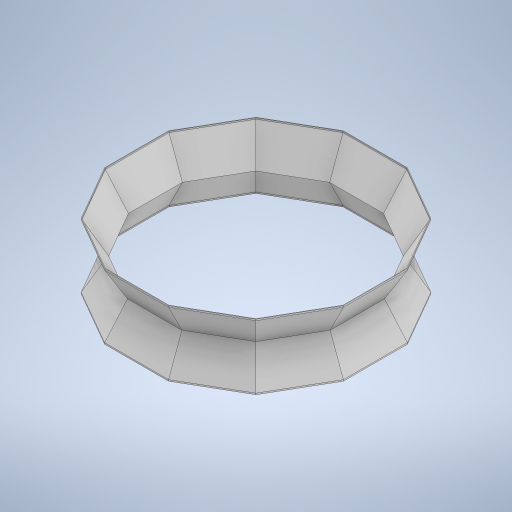
# Autodesk Inventor part: OV-PAM_n_12_standard_1F
Saved by Autodesk Inventor 2024 (Build 280153000, 153)
## iProperties
Created: 2023-08-31
Part Number: OV-PAM_n_12_standard_1F
Material: 일반
Document SubType Name: Modeling
Designer: jsw
Density: 1 g/cm^3
Appearance: 기본값
Author: jsw
Autodesk Inventor part; units mm, degrees
ref_plane "YZ Plane" through (0, 0, 0) normal (1, 0, 0) x (0, 1, 0)
ref_plane "XZ Plane" through (0, 0, 0) normal (0, 1, 0) x (-1, 0, 0)
ref_plane "XY Plane" through (0, 0, 0) normal (0, 0, 1) x (1, 0, 0)
sketch "스케치1" plane through (0, 0, 0) normal (0, 1, 0) x (-1, 0, 0)
  line L0 (-27.3911, 102.2249) -> (27.3911, 102.2249)
  line L1 (27.3911, 102.2249) -> (74.8338, 74.8338)
  line L2 (74.8338, 74.8338) -> (102.2249, 27.3911)
  line L3 (102.2249, 27.3911) -> (102.2249, -27.3911)
  line L4 (102.2249, -27.3911) -> (74.8338, -74.8338)
  line L5 (74.8338, -74.8338) -> (27.3911, -102.2249)
  line L6 (27.3911, -102.2249) -> (-27.3911, -102.2249)
  line L7 (-27.3911, -102.2249) -> (-74.8338, -74.8338)
  line L8 (-74.8338, -74.8338) -> (-102.2249, -27.3911)
  line L9 (-102.2249, -27.3911) -> (-102.2249, 27.3911)
  line L10 (-102.2249, 27.3911) -> (-74.8338, 74.8338)
  line L11 (-74.8338, 74.8338) -> (-27.3911, 102.2249)
  line L12 (27.5518, -102.8249) -> (-27.5518, -102.8249)
  line L13 (-27.5518, -102.8249) -> (-75.273, -75.273)
  line L14 (-75.273, -75.273) -> (-102.8249, -27.5518)
  line L15 (-102.8249, -27.5518) -> (-102.8249, 27.5518)
  line L16 (-102.8249, 27.5518) -> (-75.273, 75.273)
  line L17 (-75.273, 75.273) -> (-27.5518, 102.8249)
  line L18 (-27.5518, 102.8249) -> (27.5518, 102.8249)
  line L19 (27.5518, 102.8249) -> (75.273, 75.273)
  line L20 (75.273, 75.273) -> (102.8249, 27.5518)
  line L21 (102.8249, 27.5518) -> (102.8249, -27.5518)
  line L22 (102.8249, -27.5518) -> (75.273, -75.273)
  line L23 (75.273, -75.273) -> (27.5518, -102.8249)
  point P0 (0, 0)
  point P1 (0, 0)
  point P2 (0, 0)
  dimension "d1" = 211.662
  dimension "d2" = 0.6
  constraints: 48 end point, 2 coincident, 2 horizontal, 50 other
  measures "d1" distance of L8.end L2.end
  measures "d2" distance between parallel lines of L3 L21
extrude "돌출1" add sketch "스케치1" along normal blind 27 contours L0 L1 L2 L3 L4 L5 L6 L7 L8 L9 L10 L11 | L12 L13 L14 L15 L16 L17 L18 L19 L20 L21 L22 L23
ref_plane "작업 평면1" through (75.273, 0, 75.273) normal (-0.75, -0.5, -0.4330127) x (0.5, 0, -0.8660254)
sketch "스케치2" plane through (102.8249, 0, 27.5518) normal (0.8660254, 0, 0.5) x (0.5, 0, -0.8660254)
  line L0 (-55.1037, 0) -> (0, 0) projected
  line L1 (0, 0) -> (0, 27) projected
  line L2 (-55.1037, 27) -> (0, 27) projected
  line L3 (-55.1037, 0) -> (-55.1037, 27) projected
  line L4 (-55.1037, 0) -> (-102.8249, 0) projected
  line L5 (-55.1037, 0) -> (-101.8691, 27)
  line L6 (-55.1037, 27) -> (-102.8249, 27) projected
  line L7 (0, 0) -> (-1, 27)
  line L8 (-55.1037, 27) -> (-101.8691, 27)
  point P0 (-27.5518, 0)
  point P1 (-34.675, 12)
  dimension "d6" = 150
  dimension "d7" = 1
  constraints: 6 end point, 2 point on line, 1 collinear
  measures "d6" angle of L5 L0
  measures "d7" distance of L1.end L7.end
extrude "돌출2" cut sketch "스케치2" along normal up to surface surface through (75.273, 0, 75.273) normal (-0.75, -0.5, -0.4330127)
pattern_circular "원형 패턴1" count 12 over 360 about axis through (0, -10, 0) along (0, 1, 0) of "돌출2"
sketch "스케치3" plane through (0, 0, 0) normal (0, -1, 0) x (1, 0, 0)
  line L0 (-75.273, -75.273) -> (-102.8249, -27.5518) projected
  line L1 (-27.5518, -102.8249) -> (-75.273, -75.273) projected
  line L2 (27.5518, -102.8249) -> (-27.5518, -102.8249) projected
  line L3 (75.273, -75.273) -> (27.5518, -102.8249) projected
  line L4 (102.8249, -27.5518) -> (75.273, -75.273) projected
  line L5 (102.8249, 27.5518) -> (102.8249, -27.5518) projected
  line L6 (75.273, 75.273) -> (102.8249, 27.5518) projected
  line L7 (27.5518, 102.8249) -> (75.273, 75.273) projected
  line L8 (-27.5518, 102.8249) -> (27.5518, 102.8249) projected
  line L9 (-75.273, 75.273) -> (-27.5518, 102.8249) projected
  line L10 (-102.8249, 27.5518) -> (-75.273, 75.273) projected
  line L11 (-102.8249, -27.5518) -> (-102.8249, 27.5518) projected
  point P0 (0, 0)
extrude "돌출3" add sketch "스케치3" along normal blind 1.2
ref_plane "작업 평면2" through (0, 27, 0) normal (0, 1, 0) x (1, 0, 0)
mirror "미러1" about plane through (0, 27, 0) normal (0, 1, 0) of "돌출2", "원형 패턴1", "돌출3", "돌출1"
shell "쉘1" thickness 0.5 removed faces 2 at (-9.1839, 55.2, -34.275) at (-9.1839, -1.2, -34.275)
